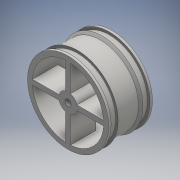
# Autodesk Inventor part: OSV Specific Wheel
Saved by Autodesk Inventor 2016 (Build 200138000, 138)
## iProperties
Created: 2016-04-05
Part Number: OSV Specific Wheel
Material: Generic
Document SubType Name: Modeling
Designer: Kenneth Daniel
Density: 1 g/cm^3
Appearance: Default
Author: Kenneth Daniel
Autodesk Inventor part; units mm, degrees
ref_plane "YZ Plane" through (0, 0, 0) normal (1, 0, 0) x (0, 1, 0)
ref_plane "XZ Plane" through (0, 0, 0) normal (0, 1, 0) x (-1, 0, 0)
ref_plane "XY Plane" through (0, 0, 0) normal (0, 0, 1) x (1, 0, 0)
sketch "Sketch1" plane through (0, 0, 0) normal (0, 0, 1) x (1, 0, 0)
  line L0 (0, 0) -> (30.65, 0)
  line L1 (30.65, 0) -> (30.65, 17.65)
  line L2 (30.65, 0) -> (30.65, 10)
  line L3 (30.65, 17.65) -> (32.65, 17.65)
  line L4 (32.65, 17.65) -> (32.65, 15.65)
  line L5 (32.65, 15.65) -> (30.65, 15.65)
  line L6 (30.65, 10) -> (32.65, 10)
  line L7 (32.65, 10) -> (30.65, 8.4317)
  line L8 (30.65, 0) -> (30.65, -17.65)
  line L9 (30.65, -17.65) -> (32.65, -17.65)
  line L10 (32.65, -17.65) -> (32.65, -15.65)
  line L11 (32.65, -15.65) -> (30.65, -15.65)
  line L12 (30.65, -10) -> (32.65, -10)
  line L13 (30.65, 17.65) -> (28.65, 17.65)
  line L14 (28.65, 17.65) -> (28.65, -17.65)
  line L15 (28.65, -17.65) -> (30.65, -17.65)
  line L16 (32.65, -10) -> (30.65, -8.6227)
  line L17 (0, -24.71) -> (0, 24.71) projected
  dimension "d1" = 30.65
  dimension "d5" = 10
  dimension "d9" = 2
  dimension "d10" = 2
  dimension "d11" = 2
  dimension "d12" = 2
  constraints: 34 end point, 6 point on line, 6 symmetric about line, 4 horizontal, 4 perpendicular, 1 parallel
  measures "d1" distance of L0.start L0.end
  measures "d5" distance of L0.end L2.end
  measures "d9" distance of L1.end L3.end
  measures "d10" distance of L3.end L4.end
  measures "d11" distance of L2.end L6.end
  measures "d12" distance of L1.end L13.end
revolve "Revolution1" add sketch "Sketch1" angle 360 about axis through (0, -10, 0) along (0, 1, 0)
sketch "Sketch2" plane through (0, 17.65, 0) normal (0, 1, 0) x (1, 0, 0)
  circle A0 centre (0, 0) radius 28.65
  circle A1 centre (0, 0) radius 7.5
  circle A2 centre (0, 0) radius 28.65 projected
  line L0 (-7.2284, -2) -> (-28.5801, -2)
  line L1 (-38.7788, 0) -> (46.3448, 0) construction
  line L2 (-7.2284, 2) -> (-28.5801, 2)
  line L3 (-7.2284, -2) -> (-7.2284, 2) construction
  line L4 (-7.2284, 2) -> (-29.2518, 2) construction
  line L5 (-29.2518, 2) -> (-29.2518, -2) construction
  line L6 (-29.2518, -2) -> (-7.2284, -2) construction
  line L7 (-7.2284, -2) -> (-7.2284, 2)
  line L8 (-7.2284, 2) -> (-29.2518, 2)
  line L9 (-29.2518, 2) -> (-29.2518, -2)
  line L10 (-29.2518, -2) -> (-7.2284, -2)
  circle A3 centre (0, 0) radius 2.5
  dimension "d14" = 15
  dimension "d16" = 5
  constraints: 22 end point, 4 parallel, 3 centre point, 3 coincident, 3 perpendicular, 2 horizontal, 2 point on circle, 1 symmetric about line, 1 vertical, 2 other
  measures "d14" diameter of A1
  measures "d16" diameter of A3
extrude "Extrusion1" add sketch "Sketch2" against normal up to surface (35.3 mm away) contours L2 A1 L0 A0 | A0 L10 L9 L8 | A1 L7 picked at (-14.5272, 0.2224) picked at (-5.6523, 0)
pattern_circular "Circular Pattern1" count 4 over 360 about axis through (0, 17.65, 0) along (0, -1, 0) of "Extrusion1"
sketch "Sketch3" plane through (0, 17.65, 0) normal (0, 1, 0) x (1, 0, 0)
  circle A0 centre (0, 0) radius 2.5 projected
  circle A1 centre (0, 0) radius 28.65
  constraints: 1 centre point, 1 coincident
extrude "Extrusion2" cut sketch "Sketch3" against normal blind 15
body "Solid1"
